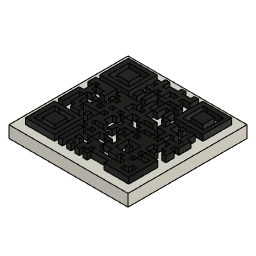
QRCoaster v2 (Autodesk Fusion 360 design; units mm, degrees)
Autodesk Fusion 360 part; units mm, degrees
sketch "Sketch1" plane through (0, 0, 0) normal (0, 0, 1) x (1, 0, 0)
  line L0 (-9.0751, 9.5831) -> (10.9249, 9.5831)
  line L1 (10.9249, 9.5831) -> (10.9249, -10.4169)
  line L2 (10.9249, -10.4169) -> (-9.0751, -10.4169)
  line L3 (-9.0751, -10.4169) -> (-9.0751, 9.5831)
  dimension "d1" = 20
  dimension "d2" = 20
  constraint horizontal L0
  constraint vertical L1
  constraint horizontal L2
  constraint vertical L3
  measures "d1" distance of L0.start L0.end
  measures "d2" distance of L0.start L2.end
extrude "Extrude1" add sketch "Sketch1" along normal blind 2 makes body 1
sketch "Sketch2" plane through (0, 0, 0) normal (0, 0, 1) x (1, 0, 0)
sketch "Sketch3" plane through (0, 0, 2) normal (0, 0, 1) x (-1, 0, 0)
  line L0 (9.0751, 10.4169) -> (-10.9249, 10.4169)
  line L1 (-10.9249, 10.4169) -> (-10.9249, -9.5831)
  line L2 (-10.9249, -9.5831) -> (9.0751, -9.5831)
  line L3 (9.0751, -9.5831) -> (9.0751, 10.4169)
  line L4 (7.7081, -8.2836) -> (-9.6385, -8.2836)
  line L5 (-9.6385, -8.2836) -> (-9.6385, 9.0072)
  line L6 (-9.6385, 9.0072) -> (7.7081, 9.0072)
  line L7 (7.7081, 9.0072) -> (7.7081, -8.2836)
  constraint horizontal L4
  constraint vertical L5
  constraint horizontal L6
  constraint vertical L7
extrude "Extrude2" add sketch "Sketch3" along normal blind 1 contours L4 L5 L6 L7 bodies 1
sketch "Sketch4" plane through (0, 0, 3) normal (0, 0, 1) x (-1, 0, 0)
  line L0 (7.7081, 9.0072) -> (-9.6385, 9.0072)
  line L1 (-9.6385, 9.0072) -> (-9.6385, -8.2836)
  line L2 (-9.6385, -8.2836) -> (7.7081, -8.2836)
  line L3 (7.7081, -8.2836) -> (7.7081, 9.0072)
  line L4 (6.9849, -7.6381) -> (3.5168, -7.6381)
  line L5 (3.5168, -7.6381) -> (3.5168, -4.1433)
  line L6 (3.5168, -4.1433) -> (6.9849, -4.1433)
  line L7 (6.9849, -4.1433) -> (6.9849, -7.6381)
  line L8 (2.8498, -8.2836) -> (2.1295, -8.2836)
  line L9 (2.1295, -8.2836) -> (2.1295, -2.8094)
  line L10 (2.1295, -2.8094) -> (2.8498, -2.8094)
  line L11 (2.8498, -2.8094) -> (2.8498, -8.2836)
  line L12 (2.1295, -8.2836) -> (1.4892, -8.2836)
  line L13 (1.4892, -8.2836) -> (1.4892, -7.6114)
  line L14 (1.4892, -7.6114) -> (2.1295, -7.6114)
  line L15 (2.1295, -7.6114) -> (2.1295, -8.2836)
  line L16 (2.1295, -6.9445) -> (1.4892, -6.9445)
  line L17 (1.4892, -6.9445) -> (1.4892, -6.2509)
  line L18 (1.4892, -6.2509) -> (2.1295, -6.2509)
  line L19 (2.1295, -6.2509) -> (2.1295, -6.9445)
  line L20 (2.1295, -5.5465) -> (0.7956, -5.5465)
  line L21 (0.7956, -5.5465) -> (0.7956, -4.8103)
  line L22 (0.7956, -4.8103) -> (2.1295, -4.8103)
  line L23 (2.1295, -4.8103) -> (2.1295, -5.5465)
  line L24 (1.4626, -4.8103) -> (0.7956, -4.8103)
  line L25 (0.7956, -4.8103) -> (0.7956, -2.7827)
  line L26 (0.7956, -2.7827) -> (1.4626, -2.7827)
  line L27 (1.4626, -2.7827) -> (1.4626, -4.8103)
  line L28 (2.1295, -3.4497) -> (1.4626, -3.4497)
  line L29 (1.4626, -3.4497) -> (1.4626, -2.7827)
  line L30 (1.4626, -2.7827) -> (2.1295, -2.7827)
  line L31 (2.1295, -2.7827) -> (2.1295, -3.4497)
  line L32 (0.7956, -3.503) -> (-0.5916, -3.503)
  line L33 (-0.5916, -3.503) -> (-0.5916, -2.7827)
  line L34 (-0.5916, -2.7827) -> (0.7956, -2.7827)
  line L35 (0.7956, -2.7827) -> (0.7956, -3.503)
  line L36 (-0.5916, -3.503) -> (0.102, -3.503)
  line L37 (0.102, -3.503) -> (0.102, -5.5306)
  line L38 (0.102, -5.5306) -> (-0.5916, -5.5306)
  line L39 (-0.5916, -5.5306) -> (-0.5916, -3.503)
  line L40 (0.102, -5.5306) -> (0.7422, -5.5306)
  line L41 (0.7422, -5.5306) -> (0.7422, -6.2509)
  line L42 (0.7422, -6.2509) -> (0.102, -6.2509)
  line L43 (0.102, -6.2509) -> (0.102, -5.5306)
  line L44 (0.7422, -7.0245) -> (0.102, -7.0245)
  line L45 (0.102, -7.0245) -> (0.102, -8.2836)
  line L46 (0.102, -8.2836) -> (0.7422, -8.2836)
  line L47 (0.7422, -8.2836) -> (0.7422, -7.0245)
  line L48 (0.102, -8.2836) -> (-1.2586, -8.2836)
  line L49 (-1.2586, -8.2836) -> (-1.2586, -7.6541)
  line L50 (-1.2586, -7.6541) -> (0.102, -7.6541)
  line L51 (0.102, -7.6541) -> (0.102, -8.2836)
  line L52 (-1.9789, -7.6541) -> (-3.3662, -7.6541)
  line L53 (-3.3662, -7.6541) -> (-3.3662, -8.2836)
  line L54 (-3.3662, -8.2836) -> (-1.9789, -8.2836)
  line L55 (-1.9789, -8.2836) -> (-1.9789, -7.6541)
  line L56 (-4.0865, -8.2836) -> (-4.7801, -8.2836)
  line L57 (-4.7801, -8.2836) -> (-4.7801, -2.8094)
  line L58 (-4.7801, -2.8094) -> (-4.0865, -2.8094)
  line L59 (-4.0865, -2.8094) -> (-4.0865, -8.2836)
  line L60 (-0.6717, -6.9178) -> (-2.0323, -6.9178)
  line L61 (-2.0323, -6.9178) -> (-2.0323, -6.2775)
  line L62 (-2.0323, -6.2775) -> (-0.6717, -6.2775)
  line L63 (-0.6717, -6.2775) -> (-0.6717, -6.9178)
  line L64 (-1.352, -5.5465) -> (-0.6717, -5.5465)
  line L65 (-0.6717, -5.5465) -> (-0.6717, -6.2775)
  line L66 (-0.6717, -6.2775) -> (-1.352, -6.2775)
  line L67 (-1.352, -6.2775) -> (-1.352, -5.5465)
  line L68 (-2.7526, -6.8911) -> (-4.0865, -6.8911)
  line L69 (-4.0865, -6.8911) -> (-4.0865, -6.2775)
  line L70 (-4.0865, -6.2775) -> (-2.7526, -6.2775)
  line L71 (-2.7526, -6.2775) -> (-2.7526, -6.8911)
  line L72 (-3.4195, -6.2775) -> (-4.0865, -6.2775)
  line L73 (-4.0865, -6.2775) -> (-4.0865, -5.5465)
  line L74 (-4.0865, -5.5465) -> (-3.4195, -5.5465)
  line L75 (-3.4195, -5.5465) -> (-3.4195, -6.2775)
  line L76 (-3.4195, -4.8636) -> (-4.0865, -4.8636)
  line L77 (-4.0865, -4.8636) -> (-4.0865, -4.2233)
  line L78 (-4.0865, -4.2233) -> (-3.4195, -4.2233)
  line L79 (-3.4195, -4.2233) -> (-3.4195, -4.8636)
  line L80 (-1.9789, -5.5465) -> (-3.4195, -5.5465)
  line L81 (-3.4195, -5.5465) -> (-3.4195, -4.8636)
  line L82 (-3.4195, -4.8636) -> (-1.9789, -4.8636)
  line L83 (-1.9789, -4.8636) -> (-1.9789, -5.5465)
  line L84 (-0.5916, -4.8636) -> (-1.9789, -4.8636)
  line L85 (-1.9789, -4.8636) -> (-1.9789, -4.2233)
  line L86 (-1.9789, -4.2233) -> (-0.5916, -4.2233)
  line L87 (-0.5916, -4.2233) -> (-0.5916, -4.8636)
  line L88 (-1.2853, -4.2233) -> (-1.9789, -4.2233)
  line L89 (-1.9789, -4.2233) -> (-1.9789, -2.7827)
  line L90 (-1.9789, -2.7827) -> (-1.2853, -2.7827)
  line L91 (-1.2853, -2.7827) -> (-1.2853, -4.2233)
  line L92 (-1.9789, -2.7827) -> (-4.0598, -2.7827)
  line L93 (-4.0598, -2.7827) -> (-4.0598, -1.3688)
  line L94 (-4.0598, -1.3688) -> (-1.9789, -1.3688)
  line L95 (-1.9789, -1.3688) -> (-1.9789, -2.7827)
  line L96 (-2.6458, -4.2233) -> (-3.4195, -4.2233)
  line L97 (-3.4195, -4.2233) -> (-3.4195, -2.7827)
  line L98 (-3.4195, -2.7827) -> (-2.6458, -2.7827)
  line L99 (-2.6458, -2.7827) -> (-2.6458, -4.2233)
  line L100 (-1.3386, -1.4755) -> (0.7689, -1.4755)
  line L101 (0.7689, -1.4755) -> (0.7689, -2.0758)
  line L102 (0.7689, -2.0758) -> (-1.3386, -2.0758)
  line L103 (-1.3386, -2.0758) -> (-1.3386, -1.4755)
  line L104 (0.0486, -2.0758) -> (-0.5916, -2.0758)
  line L105 (-0.5916, -2.0758) -> (-0.5916, -2.7827)
  line L106 (-0.5916, -2.7827) -> (0.0486, -2.7827)
  line L107 (0.0486, -2.7827) -> (0.0486, -2.0758)
  line L108 (0.0486, -0.6752) -> (0.7689, -0.6752)
  line L109 (0.7689, -0.6752) -> (0.7689, -1.4755)
  line L110 (0.7689, -1.4755) -> (0.0486, -1.4755)
  line L111 (0.0486, -1.4755) -> (0.0486, -0.6752)
  line L112 (7.7081, -3.4764) -> (2.8498, -3.4764)
  line L113 (2.8498, -3.4764) -> (2.8498, -2.8094)
  line L114 (2.8498, -2.8094) -> (7.7081, -2.8094)
  line L115 (7.7081, -2.8094) -> (7.7081, -3.4764)
  line L116 (4.2104, -2.8094) -> (3.5434, -2.8094)
  line L117 (3.5434, -2.8094) -> (3.5434, 0.6054)
  line L118 (3.5434, 0.6054) -> (4.2104, 0.6054)
  line L119 (4.2104, 0.6054) -> (4.2104, -2.8094)
  line L120 (3.5434, -2.0624) -> (2.8498, -2.0624)
  line L121 (2.8498, -2.0624) -> (2.8498, -1.4755)
  line L122 (2.8498, -1.4755) -> (3.5434, -1.4755)
  line L123 (3.5434, -1.4755) -> (3.5434, -2.0624)
  line L124 (2.1562, -0.7552) -> (2.8498, -0.7552)
  line L125 (2.8498, -0.7552) -> (2.8498, -1.4755)
  line L126 (2.8498, -1.4755) -> (2.1562, -1.4755)
  line L127 (2.1562, -1.4755) -> (2.1562, -0.7552)
  line L128 (2.8498, 0.0451) -> (3.5434, 0.0451)
  line L129 (3.5434, 0.0451) -> (3.5434, -0.7285)
  line L130 (3.5434, -0.7285) -> (2.8498, -0.7285)
  line L131 (2.8498, -0.7285) -> (2.8498, 0.0451)
  line L132 (6.9315, -2.0624) -> (6.3179, -2.0624)
  line L133 (6.3179, -2.0624) -> (6.3179, -1.4755)
  line L134 (6.3179, -1.4755) -> (6.9315, -1.4755)
  line L135 (6.9315, -1.4755) -> (6.9315, -2.0624)
  line L136 (7.7081, -1.4755) -> (6.9315, -1.4755)
  line L137 (6.9315, -1.4755) -> (6.9315, -0.0082)
  line L138 (6.9315, -0.0082) -> (7.7081, -0.0082)
  line L139 (7.7081, -0.0082) -> (7.7081, -1.4755)
  line L140 (6.3179, -1.4755) -> (4.9574, -1.4755)
  line L141 (4.9574, -1.4755) -> (4.9574, -0.7419)
  line L142 (4.9574, -0.7419) -> (6.3179, -0.7419)
  line L143 (6.3179, -0.7419) -> (6.3179, -1.4755)
  line L144 (5.6376, -0.7419) -> (4.2104, -0.7419)
  line L145 (4.2104, -0.7419) -> (4.2104, -0.0082)
  line L146 (4.2104, -0.0082) -> (5.6376, -0.0082)
  line L147 (5.6376, -0.0082) -> (5.6376, -0.7419)
  line L148 (6.3179, -0.0082) -> (4.924, -0.0082)
  line L149 (4.924, -0.0082) -> (4.924, 0.632)
  line L150 (4.924, 0.632) -> (6.3179, 0.632)
  line L151 (6.3179, 0.632) -> (6.3179, -0.0082)
  line L152 (5.621, 0.632) -> (4.2104, 0.632)
  line L153 (4.2104, 0.632) -> (4.2104, 1.3523)
  line L154 (4.2104, 1.3523) -> (5.621, 1.3523)
  line L155 (5.621, 1.3523) -> (5.621, 0.632)
  line L156 (3.5434, 0.6054) -> (2.7964, 0.6054)
  line L157 (2.7964, 0.6054) -> (2.7964, 1.3523)
  line L158 (2.7964, 1.3523) -> (3.5434, 1.3523)
  line L159 (3.5434, 1.3523) -> (3.5434, 0.6054)
  line L160 (2.1295, -0.0082) -> (1.4359, -0.0082)
  line L161 (1.4359, -0.0082) -> (1.4359, 0.6054)
  line L162 (1.4359, 0.6054) -> (2.1295, 0.6054)
  line L163 (2.1295, 0.6054) -> (2.1295, -0.0082)
  line L164 (0.7956, -0.0082) -> (0.102, -0.0082)
  line L165 (0.102, -0.0082) -> (0.102, 0.6054)
  line L166 (0.102, 0.6054) -> (0.7956, 0.6054)
  line L167 (0.7956, 0.6054) -> (0.7956, -0.0082)
  line L168 (-0.645, -0.5951) -> (-1.9522, -0.5951)
  line L169 (-1.9522, -0.5951) -> (-1.9522, 0.6054)
  line L170 (-1.9522, 0.6054) -> (-0.645, 0.6054)
  line L171 (-0.645, 0.6054) -> (-0.645, -0.5951)
  line L172 (-1.9522, 0.0051) -> (-2.6725, 0.0051)
  line L173 (-2.6725, 0.0051) -> (-2.6725, 1.3257)
  line L174 (-2.6725, 1.3257) -> (-1.9522, 1.3257)
  line L175 (-1.9522, 1.3257) -> (-1.9522, 0.0051)
  line L176 (-2.6725, 0.6654) -> (-3.3928, 0.6654)
  line L177 (-3.3928, 0.6654) -> (-3.3928, 1.3257)
  line L178 (-3.3928, 1.3257) -> (-2.6725, 1.3257)
  line L179 (-2.6725, 1.3257) -> (-2.6725, 0.6654)
  line L180 (-2.6725, -0.6752) -> (-6.194, -0.6752)
  line L181 (-6.194, -0.6752) -> (-6.194, -0.0082)
  line L182 (-6.194, -0.0082) -> (-2.6725, -0.0082)
  line L183 (-2.6725, -0.0082) -> (-2.6725, -0.6752)
  line L184 (-4.0598, -2.0758) -> (-4.7801, -2.0758)
  line L185 (-4.7801, -2.0758) -> (-4.7801, -0.6752)
  line L186 (-4.7801, -0.6752) -> (-4.0598, -0.6752)
  line L187 (-4.0598, -0.6752) -> (-4.0598, -2.0758)
  line L188 (-4.7801, -3.4764) -> (-5.4204, -3.4764)
  line L189 (-5.4204, -3.4764) -> (-5.4204, -1.3755)
  line L190 (-5.4204, -1.3755) -> (-4.7801, -1.3755)
  line L191 (-4.7801, -1.3755) -> (-4.7801, -3.4764)
  line L192 (-5.4204, -3.4764) -> (-9.6385, -3.4764)
  line L193 (-9.6385, -3.4764) -> (-9.6385, -2.7827)
  line L194 (-9.6385, -2.7827) -> (-5.4204, -2.7827)
  line L195 (-5.4204, -2.7827) -> (-5.4204, -3.4764)
  line L196 (-6.194, -2.7827) -> (-6.861, -2.7827)
  line L197 (-6.861, -2.7827) -> (-6.861, -1.4488)
  line L198 (-6.861, -1.4488) -> (-6.194, -1.4488)
  line L199 (-6.194, -1.4488) -> (-6.194, -2.7827)
  line L200 (-6.861, -1.4488) -> (-8.3016, -1.4488)
  line L201 (-8.3016, -1.4488) -> (-8.3016, -2.1158)
  line L202 (-8.3016, -2.1158) -> (-6.861, -2.1158)
  line L203 (-6.861, -2.1158) -> (-6.861, -1.4488)
  line L204 (-8.3016, -2.1158) -> (-7.5294, -2.1158)
  line L205 (-7.5294, -2.1158) -> (-7.5294, -2.7827)
  line L206 (-7.5294, -2.7827) -> (-8.3016, -2.7827)
  line L207 (-8.3016, -2.7827) -> (-8.3016, -2.1158)
  line L208 (-9.0219, -2.7827) -> (-9.6385, -2.7827)
  line L209 (-9.6385, -2.7827) -> (-9.6385, -1.4488)
  line L210 (-9.6385, -1.4488) -> (-9.0219, -1.4488)
  line L211 (-9.0219, -1.4488) -> (-9.0219, -2.7827)
  line L212 (-9.6385, 1.379) -> (-9.0219, 1.379)
  line L213 (-9.0219, 1.379) -> (-9.0219, 0.6054)
  line L214 (-9.0219, 0.6054) -> (-9.6385, 0.6054)
  line L215 (-9.6385, 0.6054) -> (-9.6385, 1.379)
  line L216 (-9.0219, -0.0616) -> (-6.861, -0.0616)
  line L217 (-6.861, -0.0616) -> (-6.861, -0.7019)
  line L218 (-6.861, -0.7019) -> (-9.0219, -0.7019)
  line L219 (-9.0219, -0.7019) -> (-9.0219, -0.0616)
  line L220 (-7.5279, -0.7019) -> (-8.3016, -0.7019)
  line L221 (-8.3016, -0.7019) -> (-8.3016, -1.4488)
  line L222 (-8.3016, -1.4488) -> (-7.5279, -1.4488)
  line L223 (-7.5279, -1.4488) -> (-7.5279, -0.7019)
  line L224 (-7.5279, 0.6854) -> (-6.861, 0.6854)
  line L225 (-6.861, 0.6854) -> (-6.861, -0.0616)
  line L226 (-6.861, -0.0616) -> (-7.5279, -0.0616)
  line L227 (-7.5279, -0.0616) -> (-7.5279, 0.6854)
  line L228 (-7.5279, 0.6854) -> (-8.3016, 0.6854)
  line L229 (-8.3016, 0.6854) -> (-8.3016, 2.7663)
  line L230 (-8.3016, 2.7663) -> (-7.5279, 2.7663)
  line L231 (-7.5279, 2.7663) -> (-7.5279, 0.6854)
  line L232 (-6.861, 2.0726) -> (-7.5279, 2.0726)
  line L233 (-7.5279, 2.0726) -> (-7.5279, 3.4065)
  line L234 (-7.5279, 3.4065) -> (-6.861, 3.4065)
  line L235 (-6.861, 3.4065) -> (-6.861, 2.0726)
  line L236 (-8.3016, 2.0993) -> (-8.9418, 2.0993)
  line L237 (-8.9418, 2.0993) -> (-8.9418, 4.1002)
  line L238 (-8.9418, 4.1002) -> (-8.3016, 4.1002)
  line L239 (-8.3016, 4.1002) -> (-8.3016, 2.0993)
  line L240 (-8.9418, 2.7663) -> (-9.6385, 2.7663)
  line L241 (-9.6385, 2.7663) -> (-9.6385, 4.1268)
  line L242 (-9.6385, 4.1268) -> (-8.9418, 4.1268)
  line L243 (-8.9418, 4.1268) -> (-8.9418, 2.7663)
  line L244 (-8.3016, 4.1002) -> (-7.5279, 4.1002)
  line L245 (-7.5279, 4.1002) -> (-7.5279, 3.4065)
  line L246 (-7.5279, 3.4065) -> (-8.3016, 3.4065)
  line L247 (-8.3016, 3.4065) -> (-8.3016, 4.1002)
  line L248 (-7.5279, 4.7938) -> (-6.8876, 4.7938)
  line L249 (-6.8876, 4.7938) -> (-6.8876, 4.1002)
  line L250 (-6.8876, 4.1002) -> (-7.5279, 4.1002)
  line L251 (-7.5279, 4.1002) -> (-7.5279, 4.7938)
  line L252 (-7.5279, 4.7938) -> (-8.9685, 4.7938)
  line L253 (-8.9685, 4.7938) -> (-8.9685, 5.5141)
  line L254 (-8.9685, 5.5141) -> (-7.5279, 5.5141)
  line L255 (-7.5279, 5.5141) -> (-7.5279, 4.7938)
  line L256 (-7.5279, 5.5141) -> (-6.8876, 5.5141)
  line L257 (-6.8876, 5.5141) -> (-6.8876, 6.181)
  line L258 (-6.8876, 6.181) -> (-7.5279, 6.181)
  line L259 (-7.5279, 6.181) -> (-7.5279, 5.5141)
  line L260 (-8.2482, 6.9523) -> (-8.9685, 6.9523)
  line L261 (-8.9685, 6.9523) -> (-8.9685, 8.2729)
  line L262 (-8.9685, 8.2729) -> (-8.2482, 8.2729)
  line L263 (-8.2482, 8.2729) -> (-8.2482, 6.9523)
  line L264 (-8.2482, 8.2729) -> (-7.5711, 8.2729)
  line L265 (-7.5711, 8.2729) -> (-7.5711, 7.6126)
  line L266 (-7.5711, 7.6126) -> (-8.2482, 7.6126)
  line L267 (-8.2482, 7.6126) -> (-8.2482, 8.2729)
  line L268 (-4.0849, 3.4924) -> (-6.1185, 3.4924)
  line L269 (-6.1185, 3.4924) -> (-6.1185, 4.1527)
  line L270 (-6.1185, 4.1527) -> (-4.0849, 4.1527)
  line L271 (-4.0849, 4.1527) -> (-4.0849, 3.4924)
  line L272 (-6.1185, 4.1527) -> (-5.4582, 4.1527)
  line L273 (-5.4582, 4.1527) -> (-5.4582, 5.3412)
  line L274 (-5.4582, 5.3412) -> (-6.1185, 5.3412)
  line L275 (-6.1185, 5.3412) -> (-6.1185, 4.1527)
  line L276 (-4.0849, 4.1527) -> (-4.798, 4.1527)
  line L277 (-4.798, 4.1527) -> (-4.798, 5.3412)
  line L278 (-4.798, 5.3412) -> (-4.0849, 5.3412)
  line L279 (-4.0849, 5.3412) -> (-4.0849, 4.1527)
  line L280 (-4.798, 5.3412) -> (-5.4582, 5.3412)
  line L281 (-5.4582, 5.3412) -> (-5.4582, 4.747)
  line L282 (-5.4582, 4.747) -> (-4.798, 4.747)
  line L283 (-4.798, 4.747) -> (-4.798, 5.3412)
  line L284 (-4.0849, 5.6317) -> (-6.1185, 5.6317)
  line L285 (-6.1185, 5.6317) -> (-6.1185, 5.3412)
  line L286 (-6.1185, 5.3412) -> (-4.0849, 5.3412)
  line L287 (-4.0849, 5.3412) -> (-4.0849, 5.6317)
  line L288 (-5.4846, 6.181) -> (-6.1185, 6.181)
  line L289 (-6.1185, 6.181) -> (-6.1185, 7.6126)
  line L290 (-6.1185, 7.6126) -> (-5.4846, 7.6126)
  line L291 (-5.4846, 7.6126) -> (-5.4846, 6.181)
  line L292 (-6.1185, 7.6126) -> (-6.8844, 7.6126)
  line L293 (-6.8844, 7.6126) -> (-6.8844, 6.8968)
  line L294 (-6.8844, 6.8968) -> (-6.1185, 6.8968)
  line L295 (-6.1185, 6.8968) -> (-6.1185, 7.6126)
  line L296 (-5.4846, 7.6126) -> (-3.3718, 7.6126)
  line L297 (-3.3718, 7.6126) -> (-3.3718, 6.8968)
  line L298 (-3.3718, 6.8968) -> (-5.4846, 6.8968)
  line L299 (-5.4846, 6.8968) -> (-5.4846, 7.6126)
  line L300 (-4.1377, 6.8968) -> (-2.6322, 6.8968)
  line L301 (-2.6322, 6.8968) -> (-2.6322, 6.2392)
  line L302 (-2.6322, 6.2392) -> (-4.1377, 6.2392)
  line L303 (-4.1377, 6.2392) -> (-4.1377, 6.8968)
  line L304 (-5.4846, 9.0072) -> (-2.6322, 9.0072)
  line L305 (-2.6322, 9.0072) -> (-2.6322, 8.3521)
  line L306 (-2.6322, 8.3521) -> (-5.4846, 8.3521)
  line L307 (-5.4846, 8.3521) -> (-5.4846, 9.0072)
  line L308 (-2.6322, 8.3521) -> (-2.0512, 8.3521)
  line L309 (-2.0512, 8.3521) -> (-2.0512, 7.5862)
  line L310 (-2.0512, 7.5862) -> (-2.6322, 7.5862)
  line L311 (-2.6322, 7.5862) -> (-2.6322, 8.3521)
  line L312 (-1.9456, 9.0072) -> (-1.3381, 9.0072)
  line L313 (-1.3381, 9.0072) -> (-1.3381, 8.3521)
  line L314 (-1.3381, 8.3521) -> (-1.9456, 8.3521)
  line L315 (-1.9456, 8.3521) -> (-1.9456, 9.0072)
  line L316 (-1.3381, 7.5862) -> (-0.5986, 7.5862)
  line L317 (-0.5986, 7.5862) -> (-0.5986, 6.9259)
  line L318 (-0.5986, 6.9259) -> (-1.3381, 6.9259)
  line L319 (-1.3381, 6.9259) -> (-1.3381, 7.5862)
  line L320 (0.0353, 6.2392) -> (-0.5986, 6.2392)
  line L321 (-0.5986, 6.2392) -> (-0.5986, 9.0072)
  line L322 (-0.5986, 9.0072) -> (0.0353, 9.0072)
  line L323 (0.0353, 9.0072) -> (0.0353, 6.2392)
  line L324 (1.4879, 5.4733) -> (0.8012, 5.4733)
  line L325 (0.8012, 5.4733) -> (0.8012, 9.0072)
  line L326 (0.8012, 9.0072) -> (1.4879, 9.0072)
  line L327 (1.4879, 9.0072) -> (1.4879, 5.4733)
  line L328 (0.8012, 6.2128) -> (0.0353, 6.2128)
  line L329 (0.0353, 6.2128) -> (0.0353, 6.9259)
  line L330 (0.0353, 6.9259) -> (0.8012, 6.9259)
  line L331 (0.8012, 6.9259) -> (0.8012, 6.2128)
  line L332 (0.8012, 7.5862) -> (0.0353, 7.5862)
  line L333 (0.0353, 7.5862) -> (0.0353, 8.3257)
  line L334 (0.0353, 8.3257) -> (0.8012, 8.3257)
  line L335 (0.8012, 8.3257) -> (0.8012, 7.5862)
  line L336 (-5.4846, -0.0082) -> (-6.1449, -0.0082)
  line L337 (-6.1449, -0.0082) -> (-6.1449, 0.7193)
  line L338 (-6.1449, 0.7193) -> (-5.4846, 0.7193)
  line L339 (-5.4846, 0.7193) -> (-5.4846, -0.0082)
  line L340 (-6.1449, 0.7193) -> (-6.9109, 0.7193)
  line L341 (-6.9109, 0.7193) -> (-6.9109, 1.3531)
  line L342 (-6.9109, 1.3531) -> (-6.1449, 1.3531)
  line L343 (-6.1449, 1.3531) -> (-6.1449, 0.7193)
  line L344 (-4.032, 0.7193) -> (-5.4582, 0.7193)
  line L345 (-5.4582, 0.7193) -> (-5.4582, 1.3531)
  line L346 (-5.4582, 1.3531) -> (-4.032, 1.3531)
  line L347 (-4.032, 1.3531) -> (-4.032, 0.7193)
  line L348 (-3.3928, 1.3257) -> (-4.032, 1.3257)
  line L349 (-4.032, 1.3257) -> (-4.032, 2.0662)
  line L350 (-4.032, 2.0662) -> (-3.3928, 2.0662)
  line L351 (-3.3928, 2.0662) -> (-3.3928, 1.3257)
  line L352 (-4.0849, 2.0662) -> (-4.7451, 2.0662)
  line L353 (-4.7451, 2.0662) -> (-4.7451, 2.7265)
  line L354 (-4.7451, 2.7265) -> (-4.0849, 2.7265)
  line L355 (-4.0849, 2.7265) -> (-4.0849, 2.0662)
  line L356 (-2.0248, 2.0662) -> (-3.3982, 2.0662)
  line L357 (-3.3982, 2.0662) -> (-3.3982, 2.7265)
  line L358 (-3.3982, 2.7265) -> (-2.0248, 2.7265)
  line L359 (-2.0248, 2.7265) -> (-2.0248, 2.0662)
  line L360 (-3.3982, 3.466) -> (-2.7115, 3.466)
  line L361 (-2.7115, 3.466) -> (-2.7115, 2.7265)
  line L362 (-2.7115, 2.7265) -> (-3.3982, 2.7265)
  line L363 (-3.3982, 2.7265) -> (-3.3982, 3.466)
  line L364 (-3.3982, 5.4997) -> (-2.7115, 5.4997)
  line L365 (-2.7115, 5.4997) -> (-2.7115, 4.1263)
  line L366 (-2.7115, 4.1263) -> (-3.3982, 4.1263)
  line L367 (-3.3982, 4.1263) -> (-3.3982, 5.4997)
  line L368 (-2.6322, 6.2392) -> (-0.5986, 6.2392)
  line L369 (-0.5986, 6.2392) -> (-0.5986, 5.4997)
  line L370 (-0.5986, 5.4997) -> (-2.6322, 5.4997)
  line L371 (-2.6322, 5.4997) -> (-2.6322, 6.2392)
  line L372 (-0.5986, 5.4997) -> (-1.972, 5.4997)
  line L373 (-1.972, 5.4997) -> (-1.972, 4.8658)
  line L374 (-1.972, 4.8658) -> (-0.5986, 4.8658)
  line L375 (-0.5986, 4.8658) -> (-0.5986, 5.4997)
  line L376 (-2.7115, 4.813) -> (-1.2853, 4.813)
  line L377 (-1.2853, 4.813) -> (-1.2853, 3.466)
  line L378 (-1.2853, 3.466) -> (-2.7115, 3.466)
  line L379 (-2.7115, 3.466) -> (-2.7115, 4.813)
  line L380 (-1.2853, 3.466) -> (-2.0248, 3.466)
  line L381 (-2.0248, 3.466) -> (-2.0248, 2.7265)
  line L382 (-2.0248, 2.7265) -> (-1.2853, 2.7265)
  line L383 (-1.2853, 2.7265) -> (-1.2853, 3.466)
  line L384 (1.4879, 3.466) -> (-1.2853, 3.466)
  line L385 (-1.2853, 3.466) -> (-1.2853, 4.1395)
  line L386 (-1.2853, 4.1395) -> (1.4879, 4.1395)
  line L387 (1.4879, 4.1395) -> (1.4879, 3.466)
  line L388 (0.102, 0.6054) -> (-0.6514, 0.6054)
  line L389 (-0.6514, 0.6054) -> (-0.6514, 3.466)
  line L390 (-0.6514, 3.466) -> (0.102, 3.466)
  line L391 (0.102, 3.466) -> (0.102, 0.6054)
  line L392 (-0.6514, 1.3267) -> (-1.2853, 1.3267)
  line L393 (-1.2853, 1.3267) -> (-1.2853, 2.0662)
  line L394 (-1.2853, 2.0662) -> (-0.6514, 2.0662)
  line L395 (-0.6514, 2.0662) -> (-0.6514, 1.3267)
  line L396 (0.7484, 1.3267) -> (0.102, 1.3267)
  line L397 (0.102, 1.3267) -> (0.102, 2.7793)
  line L398 (0.102, 2.7793) -> (0.7484, 2.7793)
  line L399 (0.7484, 2.7793) -> (0.7484, 1.3267)
  line L400 (2.1482, 1.3267) -> (1.4879, 1.3267)
  line L401 (1.4879, 1.3267) -> (1.4879, 2.0662)
  line L402 (1.4879, 2.0662) -> (2.1482, 2.0662)
  line L403 (2.1482, 2.0662) -> (2.1482, 1.3267)
  line L404 (5.621, 1.3523) -> (4.9157, 1.3523)
  line L405 (4.9157, 1.3523) -> (4.9157, 2.0662)
  line L406 (4.9157, 2.0662) -> (5.621, 2.0662)
  line L407 (5.621, 2.0662) -> (5.621, 1.3523)
  line L408 (4.9157, 2.0662) -> (2.1746, 2.0662)
  line L409 (2.1746, 2.0662) -> (2.1746, 2.7529)
  line L410 (2.1746, 2.7529) -> (4.9157, 2.7529)
  line L411 (4.9157, 2.7529) -> (4.9157, 2.0662)
  line L412 (2.1746, 2.7529) -> (2.8349, 2.7529)
  line L413 (2.8349, 2.7529) -> (2.8349, 9.0072)
  line L414 (2.8349, 9.0072) -> (2.1746, 9.0072)
  line L415 (2.1746, 9.0072) -> (2.1746, 2.7529)
  line L416 (2.1746, 4.7866) -> (1.4879, 4.7866)
  line L417 (1.4879, 4.7866) -> (1.4879, 5.4733)
  line L418 (1.4879, 5.4733) -> (2.1746, 5.4733)
  line L419 (2.1746, 5.4733) -> (2.1746, 4.7866)
  line L420 (0.7748, 4.7866) -> (0.0617, 4.7866)
  line L421 (0.0617, 4.7866) -> (0.0617, 5.4733)
  line L422 (0.0617, 5.4733) -> (0.7748, 5.4733)
  line L423 (0.7748, 5.4733) -> (0.7748, 4.7866)
  line L424 (4.2082, 2.7529) -> (3.4951, 2.7529)
  line L425 (3.4951, 2.7529) -> (3.4951, 4.1263)
  line L426 (3.4951, 4.1263) -> (4.2082, 4.1263)
  line L427 (4.2082, 4.1263) -> (4.2082, 2.7529)
  line L428 (3.4951, 4.1263) -> (2.8349, 4.1263)
  line L429 (2.8349, 4.1263) -> (2.8349, 3.466)
  line L430 (2.8349, 3.466) -> (3.4951, 3.466)
  line L431 (3.4951, 3.466) -> (3.4951, 4.1263)
  line L432 (7.7081, 3.4924) -> (4.2082, 3.4924)
  line L433 (4.2082, 3.4924) -> (4.2082, 4.1263)
  line L434 (4.2082, 4.1263) -> (7.7081, 4.1263)
  line L435 (7.7081, 4.1263) -> (7.7081, 3.4924)
  line L436 (6.9814, 0.6665) -> (6.2683, 0.6665)
  line L437 (6.2683, 0.6665) -> (6.2683, 3.4924)
  line L438 (6.2683, 3.4924) -> (6.9814, 3.4924)
  line L439 (6.9814, 3.4924) -> (6.9814, 0.6665)
  line L440 (6.2683, 3.4924) -> (5.6344, 3.4924)
  line L441 (5.6344, 3.4924) -> (5.6344, 2.7529)
  line L442 (5.6344, 2.7529) -> (6.2683, 2.7529)
  line L443 (6.2683, 2.7529) -> (6.2683, 3.4924)
  line L444 (6.9814, 4.7866) -> (6.2683, 4.7866)
  line L445 (6.2683, 4.7866) -> (6.2683, 8.2729)
  line L446 (6.2683, 8.2729) -> (6.9814, 8.2729)
  line L447 (6.9814, 8.2729) -> (6.9814, 4.7866)
  line L448 (6.2683, 8.2729) -> (3.5744, 8.2729)
  line L449 (3.5744, 8.2729) -> (3.5744, 7.6126)
  line L450 (3.5744, 7.6126) -> (6.2683, 7.6126)
  line L451 (6.2683, 7.6126) -> (6.2683, 8.2729)
  line L452 (3.5744, 7.6126) -> (4.2082, 7.6126)
  line L453 (4.2082, 7.6126) -> (4.2082, 4.8394)
  line L454 (4.2082, 4.8394) -> (3.5744, 4.8394)
  line L455 (3.5744, 4.8394) -> (3.5744, 7.6126)
  line L456 (4.2082, 4.8394) -> (6.2683, 4.8394)
  line L457 (6.2683, 4.8394) -> (6.2683, 5.5261)
  line L458 (6.2683, 5.5261) -> (4.2082, 5.5261)
  line L459 (4.2082, 5.5261) -> (4.2082, 4.8394)
  line L460 (-5.5375, -7.6381) -> (-6.1977, -7.6381)
  line L461 (-6.1977, -7.6381) -> (-6.1977, -4.1668)
  line L462 (-6.1977, -4.1668) -> (-5.5375, -4.1668)
  line L463 (-5.5375, -4.1668) -> (-5.5375, -7.6381)
  line L464 (-6.1977, -4.1668) -> (-9.0237, -4.1668)
  line L465 (-9.0237, -4.1668) -> (-9.0237, -4.8799)
  line L466 (-9.0237, -4.8799) -> (-6.1977, -4.8799)
  line L467 (-6.1977, -4.8799) -> (-6.1977, -4.1668)
  line L468 (-9.0237, -4.8799) -> (-8.1786, -4.8799)
  line L469 (-8.1786, -4.8799) -> (-8.1786, -7.5738)
  line L470 (-8.1786, -7.5738) -> (-9.0237, -7.5738)
  line L471 (-9.0237, -7.5738) -> (-9.0237, -4.8799)
  line L472 (-8.1786, -7.5738) -> (-6.1977, -7.5738)
  line L473 (-6.1977, -7.5738) -> (-6.1977, -6.9135)
  line L474 (-6.1977, -6.9135) -> (-8.1786, -6.9135)
  line L475 (-8.1786, -6.9135) -> (-8.1786, -7.5738)
  constraint horizontal L4
  constraint vertical L5
  constraint horizontal L6
  constraint vertical L7
  constraint horizontal L8
  constraint vertical L9
  constraint horizontal L10
  constraint vertical L11
  constraint coincident L2 L8.start
  constraint horizontal L12
  constraint vertical L13
  constraint horizontal L14
  constraint vertical L15
  constraint horizontal L16
  constraint vertical L17
  constraint horizontal L18
  constraint vertical L19
  constraint coincident L9 L16.start
  constraint horizontal L20
  constraint vertical L21
  constraint horizontal L22
  constraint vertical L23
  constraint midpoint L9 L20.start
  constraint horizontal L24
  constraint vertical L25
  constraint horizontal L26
  constraint vertical L27
  constraint midpoint L22 L24.start
  constraint horizontal L28
  constraint vertical L29
  constraint horizontal L30
  constraint vertical L31
  constraint coincident L9 L28.start
  constraint horizontal L32
  constraint vertical L33
  constraint horizontal L34
  constraint vertical L35
  constraint coincident L25 L32.start
  constraint horizontal L36
  constraint vertical L37
  constraint horizontal L38
  constraint vertical L39
  constraint horizontal L40
  constraint vertical L41
  constraint horizontal L42
  constraint vertical L43
  constraint horizontal L44
  constraint vertical L45
  constraint horizontal L46
  constraint vertical L47
  constraint coincident L2 L45.end
  constraint horizontal L48
  constraint vertical L49
  constraint horizontal L50
  constraint vertical L51
  constraint horizontal L52
  constraint vertical L53
  constraint horizontal L54
  constraint vertical L55
  constraint coincident L2 L53.end
  constraint horizontal L56
  constraint vertical L57
  constraint horizontal L58
  constraint vertical L59
  constraint coincident L2 L56.start
  constraint horizontal L60
  constraint vertical L61
  constraint horizontal L62
  constraint vertical L63
  constraint horizontal L64
  constraint vertical L65
  constraint horizontal L66
  constraint vertical L67
  constraint horizontal L68
  constraint vertical L69
  constraint horizontal L70
  constraint vertical L71
  constraint coincident L59 L69.end
  constraint horizontal L72
  constraint vertical L73
  constraint horizontal L74
  constraint vertical L75
  constraint midpoint L59 L73.end
  constraint midpoint L70 L72.start
  constraint horizontal L76
  constraint vertical L77
  constraint horizontal L78
  constraint vertical L79
  constraint coincident L59 L77.end
  constraint horizontal L80
  constraint vertical L81
  constraint horizontal L82
  constraint vertical L83
  constraint horizontal L84
  constraint vertical L85
  constraint horizontal L86
  constraint vertical L87
  constraint coincident L39 L84.start
  constraint horizontal L88
  constraint vertical L89
  constraint horizontal L90
  constraint vertical L91
  constraint midpoint L86 L88.start
  constraint horizontal L92
  constraint vertical L93
  constraint horizontal L94
  constraint vertical L95
  constraint horizontal L96
  constraint vertical L97
  constraint horizontal L98
  constraint vertical L99
  constraint coincident L92 L97.end
  constraint horizontal L100
  constraint vertical L101
  constraint horizontal L102
  constraint vertical L103
  constraint horizontal L104
  constraint vertical L105
  constraint horizontal L106
  constraint vertical L107
  constraint coincident L102 L104.start
  constraint horizontal L108
  constraint vertical L109
  constraint horizontal L110
  constraint vertical L111
  constraint horizontal L112
  constraint vertical L113
  constraint horizontal L114
  constraint vertical L115
  constraint coincident L3 L112.start
  constraint horizontal L116
  constraint vertical L117
  constraint horizontal L118
  constraint vertical L119
  constraint coincident L114 L116.start
  constraint horizontal L120
  constraint vertical L121
  constraint horizontal L122
  constraint vertical L123
  constraint coincident L117 L120.start
  constraint horizontal L124
  constraint vertical L125
  constraint horizontal L126
  constraint vertical L127
  constraint horizontal L128
  constraint vertical L129
  constraint horizontal L130
  constraint vertical L131
  constraint coincident L117 L129.end
  constraint horizontal L132
  constraint vertical L133
  constraint horizontal L134
  constraint vertical L135
  constraint horizontal L136
  constraint vertical L137
  constraint horizontal L138
  constraint vertical L139
  constraint coincident L3 L136.start
  constraint horizontal L140
  constraint vertical L141
  constraint horizontal L142
  constraint vertical L143
  constraint horizontal L144
  constraint vertical L145
  constraint horizontal L146
  constraint vertical L147
  constraint coincident L119 L145.end
  constraint midpoint L142 L144.start
  constraint horizontal L148
  constraint vertical L149
  constraint horizontal L150
  constraint vertical L151
  constraint horizontal L152
  constraint vertical L153
  constraint horizontal L154
  constraint vertical L155
  constraint midpoint L150 L152.start
  constraint horizontal L156
  constraint vertical L157
  constraint horizontal L158
  constraint vertical L159
  constraint horizontal L160
  constraint vertical L161
  constraint horizontal L162
  constraint vertical L163
  constraint horizontal L164
  constraint vertical L165
  constraint horizontal L166
  constraint vertical L167
  constraint horizontal L168
  constraint vertical L169
  constraint horizontal L170
  constraint vertical L171
  constraint horizontal L172
  constraint vertical L173
  constraint horizontal L174
  constraint vertical L175
  constraint midpoint L169 L172.start
  constraint horizontal L176
  constraint vertical L177
  constraint horizontal L178
  constraint vertical L179
  constraint midpoint L173 L176.start
  constraint horizontal L180
  constraint vertical L181
  constraint horizontal L182
  constraint vertical L183
  constraint horizontal L184
  constraint vertical L185
  constraint horizontal L186
  constraint vertical L187
  constraint coincident L180 L185.end
  constraint midpoint L93 L184.start
  constraint horizontal L188
  constraint vertical L189
  constraint horizontal L190
  constraint vertical L191
  constraint coincident L57 L188.start
  constraint horizontal L192
  constraint vertical L193
  constraint horizontal L194
  constraint vertical L195
  constraint coincident L1 L193.end
  constraint horizontal L196
  constraint vertical L197
  constraint horizontal L198
  constraint vertical L199
  constraint coincident L194 L196.start
  constraint horizontal L200
  constraint vertical L201
  constraint horizontal L202
  constraint vertical L203
  constraint horizontal L204
  constraint vertical L205
  constraint horizontal L206
  constraint vertical L207
  constraint midpoint L194 L205.end
  constraint horizontal L208
  constraint vertical L209
  constraint horizontal L210
  constraint vertical L211
  constraint coincident L1 L209.end
  constraint coincident L194 L208.start
  constraint horizontal L212
  constraint vertical L213
  constraint horizontal L214
  constraint vertical L215
  constraint coincident L1 L212.start
  constraint horizontal L216
  constraint vertical L217
  constraint horizontal L218
  constraint vertical L219
  constraint horizontal L220
  constraint vertical L221
  constraint horizontal L222
  constraint vertical L223
  constraint coincident L218 L220.start
  constraint horizontal L224
  constraint vertical L225
  constraint horizontal L226
  constraint vertical L227
  constraint horizontal L228
  constraint vertical L229
  constraint horizontal L230
  constraint vertical L231
  constraint horizontal L232
  constraint vertical L233
  constraint horizontal L234
  constraint vertical L235
  constraint horizontal L236
  constraint vertical L237
  constraint horizontal L238
  constraint vertical L239
  constraint coincident L229 L236.start
  constraint horizontal L240
  constraint vertical L241
  constraint horizontal L242
  constraint vertical L243
  constraint coincident L1 L241.end
  constraint coincident L237 L240.start
  constraint horizontal L244
  constraint vertical L245
  constraint horizontal L246
  constraint vertical L247
  constraint horizontal L248
  constraint vertical L249
  constraint horizontal L250
  constraint vertical L251
  constraint horizontal L252
  constraint vertical L253
  constraint horizontal L254
  constraint vertical L255
  constraint horizontal L256
  constraint vertical L257
  constraint horizontal L258
  constraint vertical L259
  constraint horizontal L260
  constraint vertical L261
  constraint horizontal L262
  constraint vertical L263
  constraint horizontal L264
  constraint vertical L265
  constraint horizontal L266
  constraint vertical L267
  constraint horizontal L268
  constraint vertical L269
  constraint horizontal L270
  constraint vertical L271
  constraint horizontal L272
  constraint vertical L273
  constraint horizontal L274
  constraint vertical L275
  constraint horizontal L276
  constraint vertical L277
  constraint horizontal L278
  constraint vertical L279
  constraint horizontal L280
  constraint vertical L281
  constraint horizontal L282
  constraint vertical L283
  constraint midpoint L273 L281.end
  constraint horizontal L284
  constraint vertical L285
  constraint horizontal L286
  constraint vertical L287
  constraint horizontal L288
  constraint vertical L289
  constraint horizontal L290
  constraint vertical L291
  constraint horizontal L292
  constraint vertical L293
  constraint horizontal L294
  constraint vertical L295
  constraint horizontal L296
  constraint vertical L297
  constraint horizontal L298
  constraint vertical L299
  constraint horizontal L300
  constraint vertical L301
  constraint horizontal L302
  constraint vertical L303
  constraint coincident L298 L300.start
  constraint horizontal L304
  constraint vertical L305
  constraint horizontal L306
  constraint vertical L307
  constraint coincident L0 L304.start
  constraint horizontal L308
  constraint vertical L309
  constraint horizontal L310
  constraint vertical L311
  constraint horizontal L312
  constraint vertical L313
  constraint horizontal L314
  constraint vertical L315
  constraint coincident L0 L312.start
  constraint horizontal L316
  constraint vertical L317
  constraint horizontal L318
  constraint vertical L319
  constraint horizontal L320
  constraint vertical L321
  constraint horizontal L322
  constraint vertical L323
  constraint coincident L0 L321.end
  constraint horizontal L324
  constraint vertical L325
  constraint horizontal L326
  constraint vertical L327
  constraint coincident L0 L325.end
  constraint horizontal L328
  constraint vertical L329
  constraint horizontal L330
  constraint vertical L331
  constraint coincident L323 L329.end
  constraint coincident L325 L328.start
  constraint horizontal L332
  constraint vertical L333
  constraint horizontal L334
  constraint vertical L335
  constraint coincident L323 L333.end
  constraint coincident L325 L332.start
  constraint horizontal L336
  constraint vertical L337
  constraint horizontal L338
  constraint vertical L339
  constraint coincident L182 L336.start
  constraint horizontal L340
  constraint vertical L341
  constraint horizontal L342
  constraint vertical L343
  constraint horizontal L344
  constraint vertical L345
  constraint horizontal L346
  constraint vertical L347
  constraint horizontal L348
  constraint vertical L349
  constraint horizontal L350
  constraint vertical L351
  constraint horizontal L352
  constraint vertical L353
  constraint horizontal L354
  constraint vertical L355
  constraint horizontal L356
  constraint vertical L357
  constraint horizontal L358
  constraint vertical L359
  constraint horizontal L360
  constraint vertical L361
  constraint horizontal L362
  constraint vertical L363
  constraint midpoint L358 L361.end
  constraint horizontal L364
  constraint vertical L365
  constraint horizontal L366
  constraint vertical L367
  constraint horizontal L368
  constraint vertical L369
  constraint horizontal L370
  constraint vertical L371
  constraint horizontal L372
  constraint vertical L373
  constraint horizontal L374
  constraint vertical L375
  constraint horizontal L376
  constraint vertical L377
  constraint horizontal L378
  constraint vertical L379
  constraint midpoint L365 L376.start
  constraint horizontal L380
  constraint vertical L381
  constraint horizontal L382
  constraint vertical L383
  constraint horizontal L384
  constraint vertical L385
  constraint horizontal L386
  constraint vertical L387
  constraint midpoint L377 L385.end
  constraint horizontal L388
  constraint vertical L389
  constraint horizontal L390
  constraint vertical L391
  constraint coincident L384 L389.end
  constraint horizontal L392
  constraint vertical L393
  constraint horizontal L394
  constraint vertical L395
  constraint coincident L389 L392.start
  constraint horizontal L396
  constraint vertical L397
  constraint horizontal L398
  constraint vertical L399
  constraint coincident L391 L397.end
  constraint horizontal L400
  constraint vertical L401
  constraint horizontal L402
  constraint vertical L403
  constraint horizontal L404
  constraint vertical L405
  constraint horizontal L406
  constraint vertical L407
  constraint horizontal L408
  constraint vertical L409
  constraint horizontal L410
  constraint vertical L411
  constraint horizontal L412
  constraint vertical L413
  constraint horizontal L414
  constraint vertical L415
  constraint coincident L0 L413.end
  constraint horizontal L416
  constraint vertical L417
  constraint horizontal L418
  constraint vertical L419
  constraint coincident L415 L416.start
  constraint horizontal L420
  constraint vertical L421
  constraint horizontal L422
  constraint vertical L423
  constraint horizontal L424
  constraint vertical L425
  constraint horizontal L426
  constraint vertical L427
  constraint horizontal L428
  constraint vertical L429
  constraint horizontal L430
  constraint vertical L431
  constraint coincident L413 L429.end
  constraint horizontal L432
  constraint vertical L433
  constraint horizontal L434
  constraint vertical L435
  constraint coincident L3 L432.start
  constraint horizontal L436
  constraint vertical L437
  constraint horizontal L438
  constraint vertical L439
  constraint coincident L432 L437.end
  constraint horizontal L440
  constraint vertical L441
  constraint horizontal L442
  constraint vertical L443
  constraint horizontal L444
  constraint vertical L445
  constraint horizontal L446
  constraint vertical L447
  constraint horizontal L448
  constraint vertical L449
  constraint horizontal L450
  constraint vertical L451
  constraint horizontal L452
  constraint vertical L453
  constraint horizontal L454
  constraint vertical L455
  constraint horizontal L456
  constraint vertical L457
  constraint horizontal L458
  constraint vertical L459
  constraint coincident L445 L457.end
  constraint horizontal L460
  constraint vertical L461
  constraint horizontal L462
  constraint vertical L463
  constraint horizontal L464
  constraint vertical L465
  constraint horizontal L466
  constraint vertical L467
  constraint horizontal L468
  constraint vertical L469
  constraint horizontal L470
  constraint vertical L471
  constraint horizontal L472
  constraint vertical L473
  constraint horizontal L474
  constraint vertical L475
  constraint coincident L461 L473.end
extrude "Extrude3" cut sketch "Sketch4" against normal blind 1 contours L0 L410 L412 L413 L414 L415 L419 L429 | L3 L427 L432 L433 L434 L435 L438 L440 | L413 L425 L428 L429 L430 L431 | L410 L424 L425 L426 L427 L431 L433 | L0 L324 L325 L326 L327 L331 L335 | L415 L416 L417 L418 L419 | L3 L136 L137 L138 L139 | L432 L436 L437 L438 L439 L443 | L298 L300 L301 L302 L303 | L368 L369 L370 L371 L372 | L308 L309 L310 L311 | L256 L257 L258 L259 | L252 L253 L254 L255 | L248 L249 L250 L251 | L340 L341 L342 L343 | L124 L125 L126 L127 | L156 L157 L158 L159 | L408 L409 L410 L411 L412 L424 | L432 L437 L440 L441 L442 L443 | L0 L317 L320 L321 L322 L323 L329 L333 | L323 L325 L332 L333 L334 L335 | L3 L11 L112 L113 L114 L115 L116 | L132 L133 L134 L135 | L323 L325 L328 L329 L330 L331 | L114 L116 L117 L118 L119 L123 L129 L145 | L140 L141 L142 L143 L144 | L154 L404 L405 L406 L407 | L0 L312 L313 L314 L315 | L316 L317 L318 L319 L321 | L2 L8 L9 L10 L11 L15 L19 L23 L31 L113 | L119 L142 L144 L145 L146 L147 L148 | L150 L152 L153 L154 L155 L404 | L117 L120 L121 L122 L123 | L0 L304 L305 L306 L307 | L2 L9 L12 L13 L14 L15 | L9 L27 L28 L29 L30 L31 | L146 L148 L149 L150 L151 L152 | L370 L372 L373 L374 L375 | L40 L41 L42 L43 | L117 L128 L129 L130 L131 | L2 L44 L45 L46 L47 L51 | L9 L16 L17 L18 L19 | L9 L20 L21 L22 L23 L24 | L22 L24 L25 L26 L27 L29 L35 | L1 L237 L240 L241 L242 L243 | L291 L296 L297 L298 L299 L300 | L2 L45 L48 L49 L50 L51 | L25 L32 L33 L34 L35 L36 L106 | L288 L289 L290 L291 L295 L299 | L34 L102 L104 L105 L106 L107 | L1 L212 L213 L214 L215 | L229 L236 L237 L238 L239 L243 L247 | L2 L52 L53 L54 L55 | L32 L36 L37 L38 L39 L87 | L100 L101 L102 L103 L104 L110 | L239 L244 L245 L246 L247 | L289 L292 L293 L294 L295 | L1 L194 L208 L209 L210 L211 | L228 L229 L230 L231 L233 L239 | L2 L56 L57 L58 L59 L69 L73 L77 L191 | L39 L84 L85 L86 L87 L88 | L100 L108 L109 L110 L111 | L1 L189 L192 L193 L194 L195 L196 L206 L208 | L231 L232 L233 L234 L235 | L59 L68 L69 L70 L71 L72 | L86 L88 L89 L90 L91 | L216 L224 L225 L226 L227 | L57 L185 L188 L189 L190 L191 L195 | L59 L70 L72 L73 L74 L75 | L80 L81 L82 L83 | L194 L202 L204 L205 L206 L207 | L216 L217 L218 L219 L220 L226 | L59 L76 L77 L78 L79 | L92 L93 L94 L95 L98 L187 | L197 L200 L201 L202 L203 L204 L222 | L93 L180 L184 L185 L186 L187 L191 | L92 L96 L97 L98 L99 | L194 L196 L197 L198 L199 L203 | L200 L218 L220 L221 L222 L223 | L180 L181 L182 L183 L186 L336 | L182 L336 L337 L338 L339 | L4 L5 L6 L7 | L60 L61 L62 L63 L66 | L62 L64 L65 L66 L67 | L160 L161 L162 L163 | L170 L384 L388 L389 L390 L391 L395 L397 | L164 L165 L166 L167 | L168 L169 L170 L171 L175 L388 | L391 L396 L397 L398 L399 | L169 L172 L173 L174 L175 L179 | L389 L392 L393 L394 L395 | L377 L384 L385 L386 L387 L390 | L173 L176 L177 L178 L179 | L365 L376 L377 L378 L379 L380 L385 | L378 L380 L381 L382 L383 | L347 L348 L349 L350 L351 L356 | L344 L345 L346 L347 L349 | L350 L356 L357 L358 L359 L362 | L358 L360 L361 L362 L363 | L364 L365 L366 L367 L379 | L260 L261 L262 L263 L267 | L263 L264 L265 L266 L267 | L268 L269 L270 L271 L272 L276 | L270 L276 L277 L278 L279 L283 L286 | L270 L272 L273 L274 L275 L281 L286 | L274 L278 L280 L284 L285 L286 L287 | L273 L277 L280 L281 L282 L283 L286 | L352 L353 L354 L355 | L400 L401 L402 L403 | L420 L421 L422 L423 | L444 L445 L446 L447 L451 L457 | L445 L453 L456 L457 L458 L459 | L445 L448 L449 L450 L451 L452 | L450 L452 L453 L454 L455 L459 | L460 L461 L462 L463 L467 L473 | L461 L469 L472 L473 L474 L475 | L461 L464 L465 L466 L467 L468 | L466 L468 L469 L470 L471 L475 bodies 1
sketch "Sketch5" plane through (0, 0, 2) normal (0, 0, 1) x (-1, 0, 0)
  line L0 (6.9849, -4.1433) -> (3.5168, -4.1433)
  line L1 (3.5168, -4.1433) -> (3.5168, -7.6381)
  line L2 (3.5168, -7.6381) -> (6.9849, -7.6381)
  line L3 (6.9849, -7.6381) -> (6.9849, -4.1433)
  line L4 (6.2753, -6.9116) -> (4.2434, -6.9116)
  line L5 (4.2434, -6.9116) -> (4.2434, -4.8966)
  line L6 (4.2434, -4.8966) -> (6.2753, -4.8966)
  line L7 (6.2753, -4.8966) -> (6.2753, -6.9116)
  constraint horizontal L4
  constraint vertical L5
  constraint horizontal L6
  constraint vertical L7
extrude "Extrude4" add sketch "Sketch5" along normal blind 1 separate body contours L4 L5 L6 L7 makes body 2
scale "Scale1" factor 0.5 about (-4.2434, 6.9116, 2) bodies 1 2
scale "Scale2" factor 0.5 about (-1.796, 3.1531, 2) bodies 2 1
